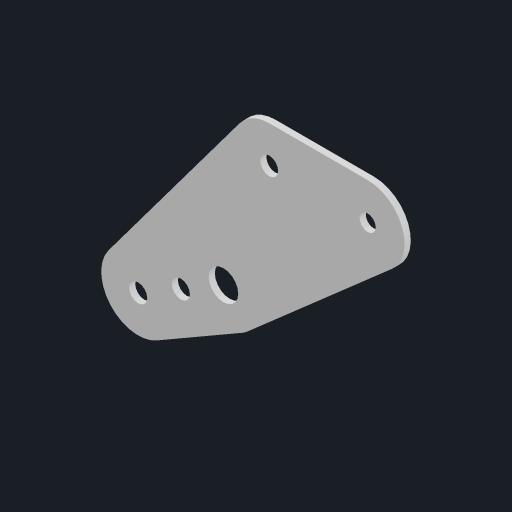
# Autodesk Inventor part: intakeMotor
Saved by Autodesk Inventor 2024.2 (Build 282272000, 272)
## iProperties
Created: 2024-01-19
Part Number: intakeMotor
Material: Generic
Document SubType Name: Modeling
Designer: reima
Density: 1 g/cm^3
Appearance: Default
Author: reima
Autodesk Inventor part; units mm, degrees
ref_plane "YZ Plane" through (0, 0, 0) normal (1, 0, 0) x (0, 1, 0)
ref_plane "XZ Plane" through (0, 0, 0) normal (0, 1, 0) x (-1, 0, 0)
ref_plane "XY Plane" through (0, 0, 0) normal (0, 0, 1) x (1, 0, 0)
sketch "Sketch1" plane through (0, 0, 0) normal (0, 0, 1) x (1, 0, 0)
  circle A0 centre (-39.737, 23.1752) radius 3 construction
  circle A1 centre (-39.737, 23.1752) radius 19.05 construction
  circle A2 centre (-7.0783, -15.7355) radius 31.75 construction
  line L0 (-66.3054, -3.825) -> (-66.3054, -14.1122) construction
  line L1 (-66.3054, -14.1122) -> (-40.9054, -14.1122) construction
  line L2 (-40.9054, -14.1122) -> (-40.9054, -3.825) construction
  line L3 (-40.9054, -3.825) -> (-66.3054, -3.825) construction
  circle A3 centre (-7.0783, -15.7355) radius 3.81
  line L4 (-7.0783, -15.7355) -> (-33.4747, -30.9755) construction
  circle A4 centre (-18.0768, -22.0855) radius 2.3368
  circle A5 centre (-29.0753, -28.4355) radius 2.3368
  circle A6 centre (4.713, 16.8252) radius 9.525
  circle A7 centre (30.113, 16.8252) radius 9.525
  circle A8 centre (-29.0753, -28.4355) radius 9.525
  circle A9 centre (-7.0783, -15.7355) radius 9.525
  line L5 (-37.7116, -24.0819) -> (-2.9197, 22.5233)
  line L6 (-24.3128, -36.6844) -> (-2.3158, -23.9844)
  line L7 (-0.804, -22.9021) -> (36.3873, 9.6587)
  line L8 (4.713, 26.3502) -> (30.113, 26.3502)
  circle A10 centre (4.713, 16.8252) radius 2.3114
  circle A11 centre (30.113, 16.8252) radius 2.0828
  point P0 (0, 0)
  point P1 (-36.708, -22.7375)
  point P2 (4.713, 26.3502)
  dimension "d1" = 63.5
  dimension "d0" = 38.1
  dimension "d2" = 25.4
  dimension "d4" = 30.48
  dimension "d5" = 4.6736
  dimension "d6" = 4.6736
  dimension "d7" = 150
  dimension "d8" = 12.7
  dimension "d9" = 12.7
  dimension "d10" = 19.05
  dimension "d11" = 19.05
  dimension "d12" = 19.05
  dimension "d13" = 19.05
  constraints: 18 end point, 11 centre point, 8 point on circle, 7 tangent, 4 coincident, 3 point on line, 2 concentric, 2 horizontal, 2 perpendicular, 5 other
  measures "d0" diameter of A1
  measures "d2" distance of L0.end L1.end
  measures "d4" distance of L4.start L4.end
  measures "d5" diameter of A4
  measures "d6" diameter of A5
  measures "d7" angle of L1 L4
  measures "d8" distance of A4.centre A5.centre
  measures "d9" distance of L4.start A4.centre
  measures "d10" diameter of A6
  measures "d11" diameter of A7
  measures "d12" diameter of A8
  measures "d13" diameter of A9
ref_plane "Work Plane1" through (0, 0, 0) normal (0, 0, -1) x (-1, 0, 0)
extrude "Extrusion2" add sketch "Sketch1" along normal blind 1.5875
body "Solid2"
